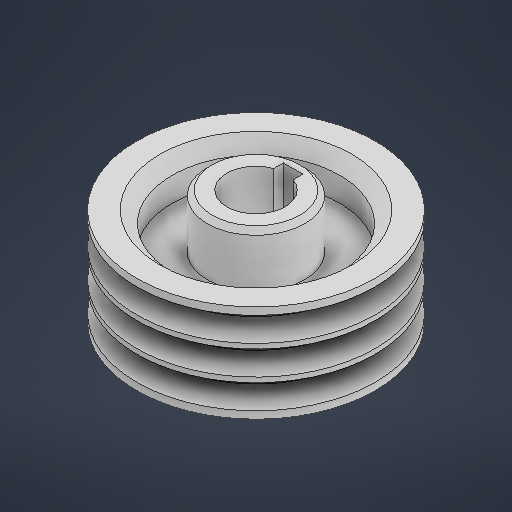
# Autodesk Inventor part: V-Belt_Pulley_3_Groove
Saved by Autodesk Inventor 2026.1 (Build 301233020, 233B)
## iProperties
Created: 2026-02-15
Part Number: V-Belt_Pulley_3_Groove
Material: Generic
Document SubType Name: Modeling
Designer: juanmiguelchungachun
Density: 1 g/cm^3
Appearance: Default
Author: juanmiguelchungachun
Autodesk Inventor part; units mm, degrees
ref_plane "YZ Plane" through (0, 0, 0) normal (1, 0, 0) x (0, 1, 0)
ref_plane "XZ Plane" through (0, 0, 0) normal (0, 1, 0) x (-1, 0, 0)
ref_plane "XY Plane" through (0, 0, 0) normal (0, 0, 1) x (1, 0, 0)
sketch "Sketch1" plane through (0, 0, 0) normal (0, 0, 1) x (1, 0, 0)
  line L0 (0, 0) -> (0, 47)
  line L1 (0, 0) -> (18, 0)
  line L2 (20, 2) -> (20, 15)
  line L3 (20, 15) -> (35, 15)
  line L4 (35, 15) -> (35, 5)
  line L5 (40, 0) -> (49, 0)
  line L6 (49, 0) -> (49, 3)
  line L7 (49, 3) -> (39.7669, 6)
  line L8 (39.7669, 6) -> (39.7669, 10)
  line L9 (39.7669, 10) -> (49, 13)
  line L10 (49, 13) -> (49, 15)
  line L11 (49, 15) -> (39.7669, 18)
  line L12 (39.7669, 18) -> (39.7669, 22)
  line L13 (39.7669, 22) -> (49, 25)
  line L14 (49, 25) -> (49, 27)
  line L15 (49, 27) -> (39.7669, 30)
  line L16 (39.7669, 30) -> (39.7669, 34)
  line L17 (39.7669, 34) -> (49, 37)
  line L18 (49, 37) -> (49, 40)
  line L19 (49, 40) -> (39.5, 40)
  line L20 (34.5, 35) -> (34.5, 25)
  line L21 (34.5, 25) -> (20, 25)
  line L22 (20, 25) -> (20, 45)
  line L23 (18, 47) -> (0, 47)
  line L24 (18, 47) -> (20, 45)
  line L25 (20, 2) -> (18, 0)
  line L26 (35, 5) -> (40, 0)
  line L27 (34.5, 35) -> (39.5, 40)
  point P0 (20, 0)
  point P1 (35, 0)
  point P2 (39.7669, 8)
  point P3 (39.7669, 20)
  point P4 (34.5, 40)
  point P5 (20, 47)
  dimension "d0" = 40
  dimension "d1" = 70
  dimension "d2" = 98
  dimension "d3" = 15
  dimension "d4" = 4
  dimension "d5" = 10
  dimension "d6" = 8
  dimension "d7" = 12
  dimension "d8" = 36
  dimension "d9" = 18
  dimension "d10" = 40
  dimension "d11" = 15
  dimension "d12" = 40
  dimension "d13" = 47
  dimension "d14" = 2
  dimension "d15" = 45
  dimension "d16" = 2
  dimension "d17" = 45
  dimension "d18" = 5
  dimension "d19" = 45
  dimension "d20" = 5
  dimension "d21" = 45
  dimension "d22" = 9.5
  constraints: 56 end point, 10 point on line, 8 collinear, 8 parallel, 7 perpendicular, 4 vertical, 2 horizontal, 2 midpoint
  measures "d0" diameter of L2 L0
  measures "d1" diameter of L4 L0
  measures "d2" diameter of L6 L0
  measures "d3" distance of point (20, 0) L2.end
  measures "d4" distance of L7.end L8.end
  measures "d5" distance of L6.end L9.end
  measures "d6" vertical distance of point (39.767, 8) L5.end
  measures "d7" distance of point (39.767, 20) point (39.767, 8)
  measures "d8" angle of L9 L7
  measures "d9" angle of L9 L5
  measures "d10" diameter of L22 L0
  measures "d11" distance of point (34.5, 40) L20.end
  measures "d12" distance between parallel lines of L19 L5
  measures "d13" distance of L0.start L0.end
  measures "d14" distance of L23.start point (20, 47)
  measures "d15" angle of L23 L24
  measures "d16" distance of L2.start point (20, 0)
  measures "d17" angle of L2 L25
  measures "d18" distance of L4.end point (35, 0)
  measures "d19" angle of L4 L26
  measures "d20" distance of L20.start point (34.5, 40)
  measures "d21" angle of L20 L27
  measures "d22" distance from line of L18 L19.end
revolve "Revolution1" add sketch "Sketch1" angle 360 about axis through (0, 0, 0) along (0, 1, 0)
sketch "Sketch2" plane through (0, 47, 0) normal (0, 1, 0) x (1, 0, 0)
  circle A0 centre (0, 0) radius 12
  line L0 (-4, 11.3137) -> (-4, 15.3)
  line L1 (-4, 15.3) -> (4, 15.3)
  line L2 (4, 15.3) -> (4, 11.3137)
  point P0 (0, -12)
  dimension "d24" = 24
  dimension "d25" = 27.3
  dimension "d26" = 8
  constraints: 6 end point, 3 point on circle, 2 perpendicular, 1 centre point, 1 coincident, 1 horizontal alignment, 1 vertical, 1 vertical alignment
  measures "d24" diameter of A0
  measures "d25" distance from line of L1 point (0, -12)
  measures "d26" distance of L0.end L1.end
extrude "Extrusion1" cut sketch "Sketch2" against normal up to surface (47 mm away)
equation "\"d9\" = 0.5 * d8"
equation "\"d16\" = d14"
equation "\"d17\" = d15"
equation "\"d20\" = d18"
equation "\"d21\" = d19"
body "Solid1"
